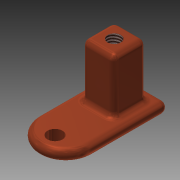
# Autodesk Inventor part: termination_lv_conductor
Saved by Autodesk Inventor 2014 SP1 (Build 180222100, 222)
## iProperties
Created: 2016-09-08
Part Number: termination_lv_conductor
Material: Copper, Cast
Document SubType Name: Modeling
Designer: tguillod
Density: 8.94 g/cm^3
Appearance: Copper - Satin
Author: tguillod
Autodesk Inventor part; units mm, degrees
ref_plane "YZ Plane" through (0, 0, 0) normal (1, 0, 0) x (0, 1, 0)
ref_plane "XZ Plane" through (0, 0, 0) normal (0, 1, 0) x (-1, 0, 0)
ref_plane "XY Plane" through (0, 0, 0) normal (0, 0, 1) x (1, 0, 0)
sketch "Sketch1" plane through (0, 0, 0) normal (0, 0, 1) x (1, 0, 0)
  line L0 (0, 0) -> (6, 0)
  line L1 (6, 0) -> (6, 6)
  line L2 (6, 6) -> (0, 6)
  line L3 (0, 6) -> (0, 0)
  dimension "d0" = 6
  dimension "d1" = 6
  constraints: 8 end point, 2 parallel, 1 horizontal, 1 perpendicular
  measures "d0" distance of L1.end L2.end
  measures "d1" distance of L0.end L1.end
extrude "Extrusion1" add sketch "Sketch1" along normal blind 10
sketch "Sketch8" plane through (0, 0, 0) normal (0, 0, -1) x (-1, 0, 0)
  line L0 (0, 0) -> (-6, 0) projected
  line L1 (0, 6) -> (0, 0) projected
  line L2 (-6, 6) -> (0, 6) projected
  line L3 (-6, 0) -> (-6, 6) projected
  line L4 (-8, 8) -> (2, 8)
  line L5 (2, 8) -> (2, -11)
  line L6 (2, -11) -> (-8, -11)
  line L7 (-8, -11) -> (-8, 8)
  dimension "d46" = 2
  dimension "d47" = 2
  dimension "d48" = 2
  dimension "d49" = 11
  constraints: 8 end point, 2 parallel, 1 horizontal, 1 perpendicular
  measures "d46" distance between parallel lines of L4 L2
  measures "d47" distance between parallel lines of L5 L1
  measures "d48" distance between parallel lines of L7 L3
  measures "d49" distance between parallel lines of L6 L0
extrude "Extrusion4" add sketch "Sketch8" along normal blind 2 contours L0 L3 L2 L1 | L4 L5 L6 L7
sketch "Sketch9" plane through (0, 0, 10) normal (0, 0, 1) x (1, 0, 0)
  line L0 (0, 6) -> (6, 0) construction
  line L1 (0, 0) -> (6, 6) construction
  point P0 (3, 3)
  constraints: 4 end point, 1 midpoint, 1 perpendicular
hole "Hole5" at (3, 3, 10) direction (0, 0, -1) diameter 2.459 depth 8 tip angle 118 thread size "M3x0.5" class "6H" standard "ISO Metric profile"
sketch "Sketch10" plane through (0, 0, 0) normal (0, 0, 1) x (1, 0, 0)
  line L0 (8, 8) -> (-2, 8) projected
  line L1 (-2, -11) -> (8, -11) projected
  line L2 (3, -11) -> (3, 8) construction
  point P0 (3, -8)
  dimension "d59" = 3
  constraints: 2 end point, 2 midpoint, 1 point on line
  measures "d59" distance from line of point (3, -8) L1
hole "Hole6" at (3, -8, 0) direction (0, 0, -1) diameter 2.8 end through all
fillet "Fillet4" radius 5 2 edges at (8, -11, -1) (-2, -11, -1)
fillet "Fillet5" radius 1 8 edges at (0, 0, 5) (0, 3, 10) (0, 6, 5) (3, 6, 10) (6, 6, 5) (6, 3, 10) (6, 0, 5) (3, 0, 10)
fillet "Fillet6" radius 1 8 edges at (3, 6, 0) (0.2929, 5.7071, 0) (0, 3, 0) (0.2929, 0.2929, 0) (3, 0, 0) (5.7071, 0.2929, 0) (6, 3, 0) (5.7071, 5.7071, 0)
fillet "Fillet8" radius 0.999 4 edges at (8, 8, -1) (-2, 8, -1) (3, 8, 0) (3, 8, -2)
fillet "Fillet9" radius 0.999 10 edges at (7.7074, 7.7074, -0.2926) (-0.5356, -9.5356, 0) (-2, 0.5005, 0) (-1.7074, 7.7074, -0.2926) (8, 0.5005, 0) (-0.5356, -9.5356, -2) (-2, 0.5005, -2) (-1.7074, 7.7074, -1.7074) (7.7074, 7.7074, -1.7074) (8, 0.5005, -2)
body "Solid1"
